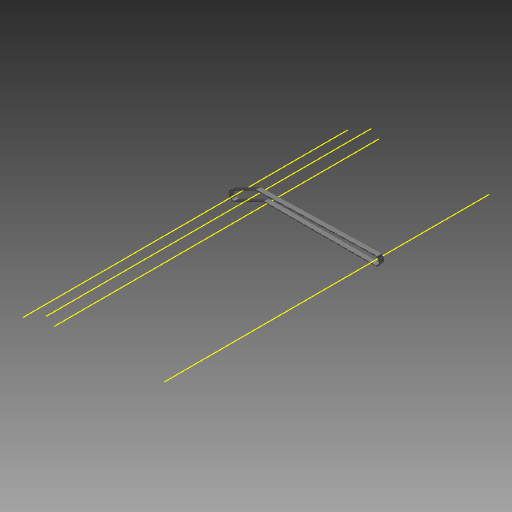
# Autodesk Inventor part: Zahnriemen
Saved by Autodesk Inventor 2019.1 (Build 231200000, 200)
## iProperties
Created: 2018-11-28
Part Number: Zahnriemen
Material: Rubber
Document SubType Name: Modeling
Designer: JochenAlt
Density: 1 g/cm^3
Appearance: Rubber - Black - Version 1.1
CustomPartVersion: 1
Author: JochenAlt
Autodesk Inventor part; units mm, degrees
sketch "Skizzenpfad" plane through (0, 0, 0) normal (0, 0, 1) x (1, 0, 0)
  arc A0 (20.91835, 14.682051) -> (19.564749, 14.341157) centre (21, 11.5) ccw
  arc A1 (127.167049, 9.449131) -> (127.059003, 17.405564) centre (127.161065, 13.428) ccw
  arc A2 (27.996541, 9.299997) -> (26.970103, 9.056529) centre (28, 7) ccw
  arc A3 (-1.794064, 3.551446) -> (1.781665, -3.557682) centre (0, 0) ccw
  line L0 (-1.794064, 3.551446) -> (19.564749, 14.341157)
  line L1 (20.91835, 14.682051) -> (127.059003, 17.405564)
  line L2 (127.167049, 9.449131) -> (27.996541, 9.299997)
  line L3 (26.970103, 9.056529) -> (1.781665, -3.557682)
  constraints: 8 end point, 8 point on circle, 4 centre point
ref_plane "Querschnittsebene" through (19.564749, 14.341157, 0) normal (-0.8925758, -0.4508975, 0) x (0, 0, 1)
ref_plane "Arbeitsebene2" through (21, 11.5, 0) normal (-1, 0, 0) x (0, 0, 1)
ref_plane "Arbeitsebene3" through (127.161065, 13.428, 0) normal (-0.9467755, 0.3218947, 0) x (0, 0, 1)
ref_plane "Arbeitsebene4" through (0, 0, 0) normal (0.9748553, 0.2228388, 0) x (0, 0, 1)
sketch "Querschnitt" plane through (19.564749, 14.341157, 0) normal (-0.8925758, -0.4508975, 0) x (0, 0, 1)
  line L0 (-2, 0.3) -> (2, 0.3)
  line L1 (2, 0.3) -> (2, -0.3)
  line L2 (2, -0.3) -> (-2, -0.3)
  line L3 (-2, -0.3) -> (-2, 0.3)
  line L4 (-2, 0) -> (2, 0) construction
  point P0 (0, 0)
  point P1 (0, 0)
  dimension "d0" = 4
  dimension "d4" = 0.3
  dimension "d5" = 0.3
  constraints: 10 end point, 3 midpoint, 2 parallel, 1 coincident, 1 horizontal, 1 perpendicular, 1 other
  measures "d0" distance between parallel lines of L1 L3
  measures "d4" distance between parallel lines of L2 L4
  measures "d5" distance between parallel lines of L4 L0
sweep "Riemen" add profiles "Querschnitt" path "Skizzenpfad"
equation "\"d0\" = da_B"
equation "\"d4\" = da_a"
equation "\"d5\" = da_a2"
equation "\"da_B\" = 4"
equation "\"da_pb\" = 2.5"
equation "\"da_L\" = 285"
equation "\"da_a\" = 0.3"
equation "\"da_S\" = 1.5"
equation "\"da_Beta\" = 20deg"
equation "\"da_Ht\" = 0.7"
equation "\"da_H\" = 1.3"
equation "\"da_a2\" = 0.3"
body "Solid1"
